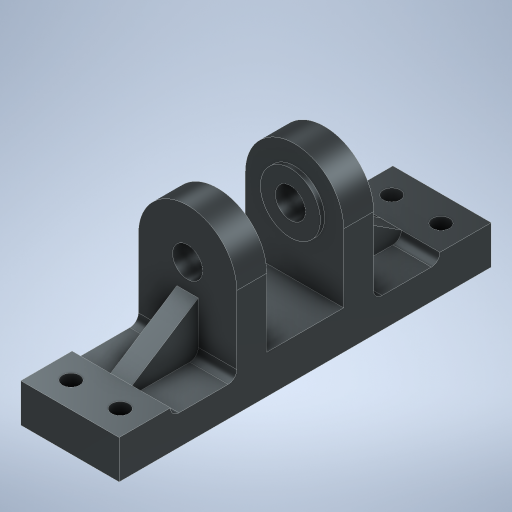
# Autodesk Inventor part: Semelle
Saved by Autodesk Inventor 2023.2 (Build 272271030, 271C)
## iProperties
Created: 2023-03-23
Part Number: Semelle
Material: Iron, Cast
Document SubType Name: Modeling
Designer: Luis Valente
Density: 7.15 g/cm^3
Appearance: Iron Gray
Author: Luis Valente
Autodesk Inventor part; units mm, degrees
ref_plane "XZ Plane" through (0, 0, 0) normal (0, 1, 0) x (-1, 0, 0)
sketch "Sketch1" plane through (0, 0, 0) normal (0, 1, 0) x (-1, 0, 0)
  line L0 (0, 0) -> (-46, 0)
  line L1 (-46, 0) -> (-46, -174)
  line L2 (-46, -174) -> (0, -174)
  line L3 (0, -174) -> (0, 0)
  dimension "d0" = 46
  dimension "d1" = 174
  constraints: 8 end point, 2 parallel, 1 horizontal, 1 perpendicular
  measures "d0" distance of L2.end L1.end
  measures "d1" distance of L1.end L0.end
extrude "Extrusion1" add sketch "Sketch1" along normal blind 18
sketch "Sketch2" plane through (0, 18, 0) normal (0, 1, 0) x (1, 0, 0)
  line L0 (0, 0) -> (0, 24)
  line L1 (0, 174) -> (0, 0) projected
  line L2 (46, 0) -> (46, 174) projected
  line L3 (0, 24) -> (46, 24)
  line L4 (46, 24) -> (46, 55)
  line L5 (46, 55) -> (0, 55)
  line L6 (0, 55) -> (0, 24)
  line L7 (0, 174) -> (0, 150)
  line L8 (0, 150) -> (46, 150)
  line L9 (46, 150) -> (46, 119)
  line L10 (46, 119) -> (0, 119)
  line L11 (0, 119) -> (0, 150)
  dimension "d4" = 24
  dimension "d5" = 31
  dimension "d6" = 24
  dimension "d7" = 31
  constraints: 20 end point, 4 parallel, 4 point on line, 2 horizontal, 2 perpendicular
  measures "d4" distance of L0.start L0.end
  measures "d5" distance of L4.end L3.end
  measures "d6" distance of L1.start L7.end
  measures "d7" distance of L8.end L9.end
extrude "Extrusion2" cut sketch "Sketch2" against normal blind 4 contours L8 L2 L10 L1 | L5 L2 L3 L1
fillet "Fillet1" radius 4 4 edges at (23, 14, -24) (23, 14, -119) (23, 14, -55) (23, 14, -150)
sketch "Sketch3" plane through (0, 18, 0) normal (0, 1, 0) x (1, 0, 0)
  line L0 (46, 150) -> (46, 174) projected
  line L1 (46, 162) -> (0, 162)
  line L2 (46, 174) -> (0, 174) projected
  line L3 (23, 174) -> (23, 150)
  line L4 (23, 174) -> (34.5, 174)
  line L5 (34.5, 174) -> (34.5, 150)
  line L6 (0, 150) -> (46, 150) projected
  line L7 (23, 174) -> (11.5, 174)
  line L8 (11.5, 174) -> (11.5, 150)
  line L9 (0, 0) -> (46, 0) projected
  line L10 (23, 0) -> (23, 24)
  line L11 (46, 24) -> (0, 24) projected
  line L12 (46, 0) -> (46, 174) projected
  line L13 (46, 12) -> (0, 12)
  line L14 (34.5, 0) -> (34.5, 24)
  line L15 (11.5, 0) -> (11.5, 24)
  circle A0 centre (34.5, 12) radius 4
  circle A1 centre (11.5, 12) radius 4
  circle A2 centre (34.5, 162) radius 4
  circle A3 centre (11.5, 162) radius 4
  dimension "d11" = 11.5
  dimension "d12" = 11.5
  dimension "d13" = 8
  dimension "d14" = 8
  dimension "d15" = 8
  dimension "d16" = 8
  constraints: 20 end point, 8 midpoint, 8 point on line, 4 centre point, 4 perpendicular, 2 horizontal, 1 vertical
  measures "d11" distance of L3.start L4.end
  measures "d12" distance of L3.start L7.end
  measures "d13" diameter of A0
  measures "d14" diameter of A1
  measures "d15" diameter of A2
  measures "d16" diameter of A3
hole "Hole1" at (34.5, 18, -12) at (11.5, 18, -12) at (34.5, 18, -162) at (11.5, 18, -162) direction (0, -1, 0) diameter 8 depth 18 tip angle 120
sketch "Sketch4" plane through (0, 18, 0) normal (0, 1, 0) x (1, 0, 0)
  line L0 (0, 55) -> (46, 55) projected
  line L1 (46, 0) -> (46, 174) projected
  line L2 (0, 55) -> (46, 55)
  line L3 (46, 55) -> (46, 69)
  line L4 (46, 69) -> (0, 69)
  line L5 (0, 69) -> (0, 55)
  line L6 (46, 119) -> (0, 119) projected
  line L7 (0, 119) -> (46, 119)
  line L8 (46, 119) -> (46, 105)
  line L9 (46, 105) -> (0, 105)
  line L10 (0, 105) -> (0, 119)
  point P0 (0, 0)
  dimension "d24" = 14
  dimension "d25" = 14
  constraints: 16 end point, 4 parallel, 2 horizontal, 2 perpendicular, 2 point on line
  measures "d24" distance of L3.end L2.end
  measures "d25" distance of L7.end L8.end
extrude "Extrusion3" add sketch "Sketch4" along normal blind 32
sketch "Sketch8" plane through (46, 18, -119) normal (0, 0, -1) x (-1, 0, 0)
  line L0 (0, 32) -> (46, 32) projected
  circle A0 centre (23, 32) radius 23
  point P0 (46, -18)
  dimension "d35" = 46
  constraints: 1 centre point, 1 midpoint
  measures "d35" diameter of A0
sketch "Sketch9" plane through (0, 18, -55) normal (0, 0, 1) x (1, 0, 0)
  line L0 (46, 32) -> (0, 32) projected
  circle A0 centre (23, 32) radius 23
  point P0 (0, -18)
  dimension "d36" = 46
  constraints: 1 centre point, 1 midpoint
  measures "d36" diameter of A0
extrude "Extrusion6" add sketch "Sketch9" against normal blind 14 contours L0 A0 picked at (25.7186, 39.1685)
extrude "Extrusion7" add sketch "Sketch8" against normal blind 14 contours A0 L0 picked at (25.7186, 39.1685)
sketch "Sketch14" plane through (46, 18, -69) normal (0, 0, -1) x (-1, 0, 0)
  line L0 (0, -18) -> (46, -18) projected
  line L1 (0, -18) -> (0, 32)
  line L2 (0, 32) -> (46, 32)
  circle A0 centre (23, 32) radius 14
  dimension "d51" = 50
  dimension "d52" = 28
  constraints: 4 end point, 1 centre point, 1 midpoint, 1 perpendicular, 1 vertical
  measures "d51" distance of L0.start L1.end
  measures "d52" diameter of A0
extrude "Extrusion10" add sketch "Sketch14" along normal blind 2
sketch "Sketch15" plane through (0, 18, -105) normal (0, 0, 1) x (1, 0, 0)
  line L0 (0, -18) -> (0, 32)
  line L1 (0, 32) -> (46.1632, 32)
  line L2 (0, -18) -> (0, 0) projected
  circle A0 centre (23.0816, 32) radius 14
  dimension "d55" = 50
  dimension "d56" = 28
  constraints: 4 end point, 1 centre point, 1 midpoint, 1 perpendicular, 1 vertical
  measures "d55" distance of L0.start L0.end
  measures "d56" diameter of A0
extrude "Extrusion11" add sketch "Sketch15" along normal blind 2
sketch "Sketch16" plane through (23, 50, -71) normal (0, 0, -1) x (-1, 0, 0)
  circle A0 centre (0, 0) radius 7
  point P0 (23, -50)
  dimension "d59" = 14
  constraints: 1 centre point
  measures "d59" diameter of A0
extrude "Extrusion12" cut sketch "Sketch16" against normal blind 16
sketch "Sketch17" plane through (23.0816, 50, -103) normal (0, 0, 1) x (1, 0, 0)
  circle A0 centre (0, 0) radius 7
  point P0 (-23.0816, -50)
  dimension "d62" = 14
  constraints: 1 centre point
  measures "d62" diameter of A0
extrude "Extrusion13" cut sketch "Sketch17" against normal blind 16
ref_plane "Work Plane1" through (23, 0, 0) normal (1, 0, 0) x (0, 1, 0)
sketch "Sketch21" plane through (23, 0, 0) normal (1, 0, 0) x (0, 1, 0)
  line L0 (18, -55) -> (50, -55) projected
  line L1 (50, -55) -> (38, -55)
  line L2 (38, -55) -> (14, -55)
  line L3 (14, -55) -> (14, -24)
  arc A0 (18, -24) -> (14, -28) centre (18, -28) ccw projected
  line L4 (14, -24) -> (18, -24)
  line L5 (18, -24) -> (38, -55)
  line L6 (14, -55) -> (38, -55)
  line L7 (18, -24) -> (14, -24)
  line L8 (14, -55) -> (14, -24)
  line L9 (18, -24) -> (14, -24)
  point P0 (0, 0)
  dimension "d73" = 12
  constraints: 18 end point, 4 perpendicular, 2 parallel, 1 horizontal, 1 point on line, 1 tangent
  measures "d73" distance of L0.end L1.end
extrude "Extrusion16" add sketch "Sketch21" along normal mid plane 10 contours L2 L3 A0 L5 L0
ref_plane "Work Plane2" through (0, 0, -87) normal (0, 0, 1) x (1, 0, 0)
mirror "Mirror1" about plane through (0, 0, -87) normal (0, 0, 1) of "Extrusion16"
body "Solid1"
